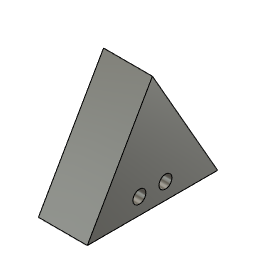
Лопатка v5 (Autodesk Fusion 360 design; units mm, degrees)
Autodesk Fusion 360 part; units mm, degrees
sketch "Sketch1" plane through (0, 0, 0) normal (1, 0, 0) x (0, 0, -1)
  line L0 (0, 0) -> (-40, 0)
  line L1 (-20, 0) -> (-20, 35)
  line L2 (-20, 35) -> (-40, 0)
  line L3 (-20, 35) -> (0, 0)
  dimension "d1" = 40
  dimension "d2" = 40.3113
  constraint coincident L0.start L3.end
  constraint horizontal L0
  constraint midpoint L0 L1.start
  constraint perpendicular L0 L1
  measures "d1" distance of L0.start L0.end
  measures "d2" distance of L1.end L0.start
extrude "Extrude1" add sketch "Sketch1" along normal blind 5
extrude "Extrude2" add 1 faces at (5, 11.6667, 26.6667) along direction (1, 0, 0) blind 10
sketch "Sketch2" plane through (15, 0, 0) normal (1, 0, 0) x (0, 0, -1)
  line L0 (-20, 35) -> (-40, 0)
  line L1 (-40, 0) -> (0, 0)
  line L2 (0, 0) -> (-20, 35)
  circle A0 centre (-24, 4.9922) radius 2
  circle A1 centre (-16, 4.9922) radius 2
  line L3 (-20, 35) -> (-20, 0)
  dimension "d7" = 4
  dimension "d8" = 4
  dimension "d9" = 4
  dimension "d10" = 4
  constraint coincident L0.start L2.end
  constraint midpoint L1 L3.end
  measures "d7" diameter of A0
  measures "d8" diameter of A1
  measures "d9" distance of A0.centre L3
  measures "d10" distance of A1.centre L3
extrude "Extrude3" cut sketch "Sketch2" against normal blind 31 contours A0 | A1
